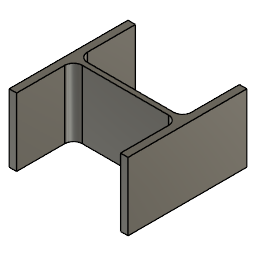
H-175×175×7.5×11 (Autodesk Fusion 360 design; units mm, degrees)
Autodesk Fusion 360 part; units mm, degrees
sketch "スケッチ1" plane through (0, 0, 0) normal (0, 0, 1) x (1, 0, 0)
  line L0 (0, 87.5) -> (0, -87.5)
  line L1 (175, -87.5) -> (175, 87.5)
  line L2 (151, 3.75) -> (24, 3.75)
  line L3 (24, -3.75) -> (151, -3.75)
  line L4 (11, -87.5) -> (11, -16.75)
  line L5 (0, -87.5) -> (11, -87.5)
  line L6 (164, -16.75) -> (164, -87.5)
  line L7 (164, -87.5) -> (175, -87.5)
  line L8 (11, 16.75) -> (11, 87.5)
  line L9 (11, 87.5) -> (0, 87.5)
  line L10 (164, 87.5) -> (164, 16.75)
  line L11 (175, 87.5) -> (164, 87.5)
  arc A0 (24, -3.75) -> (11, -16.75) centre (24, -16.75) ccw
  arc A1 (11, 16.75) -> (24, 3.75) centre (24, 16.75) ccw
  arc A2 (151, 3.75) -> (164, 16.75) centre (151, 16.75) ccw
  arc A3 (164, -16.75) -> (151, -3.75) centre (151, -16.75) ccw
extrude "押し出し1" add sketch "スケッチ1" along normal blind 100
